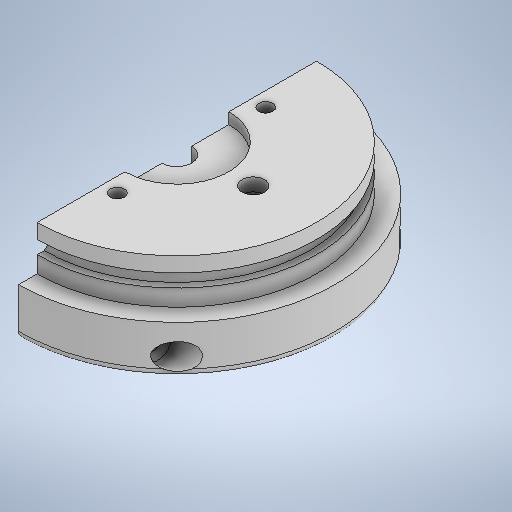
# Autodesk Inventor part: cap2_v0.7.0
Saved by Autodesk Inventor 2025 (Build 290162000, 162)
## iProperties
Created: 2026-01-07
Part Number: cap2_v0.7.0
Material: Generic
Document SubType Name: Modeling
Designer: SLM30
Density: 1 g/cm^3
Appearance: Default
Author: SLM30
Autodesk Inventor part; units mm, degrees
ref_plane "XZ Plane" through (0, 0, 0) normal (0, 1, 0) x (-1, 0, 0)
ref_plane "XY Plane" through (0, 0, 0) normal (0, 0, 1) x (1, 0, 0)
sketch "Sketch4" plane through (0, 0, 0) normal (1, 0, 0) x (0, 1, 0)
  line L0 (0, 0) -> (0, 14)
  line L1 (0, 14) -> (3, 14)
  line L2 (3, 14) -> (3, 37.65)
  line L3 (3, 37.65) -> (-9, 37.65)
  line L4 (-9, 37.65) -> (-9, 42.65)
  line L5 (0, 0) -> (-10, 0)
  line L6 (-10, 0) -> (-10, 15)
  line L7 (-10, 15) -> (-21, 15)
  line L8 (-21, 15) -> (-21, 0)
  line L9 (-21, 0) -> (-29, 0)
  line L10 (-9, 42.65) -> (-21, 42.65)
  line L11 (-21, 42.65) -> (-29, 31.0679)
  line L12 (-29, 31.0679) -> (-29, 0)
  arc A0 (-4.5225, 35.7688) -> (-0.9925, 37.65) centre (-2.7575, 36.7094) ccw
  line L13 (-4.5225, 37.65) -> (-4.5225, 35.7688)
  line L14 (-35.4, 0) -> (9.4, 0) projected
  dimension "d29" = 14
  dimension "d30" = 3
  dimension "d31" = 23.65
  dimension "d32" = 12
  dimension "d33" = 5
  dimension "d34" = 10
  dimension "d35" = 15
  dimension "d36" = 11
  dimension "d37" = 8
  dimension "d38" = 11.5821
  dimension "d39" = 124.634
  dimension "d40" = 3.53
  dimension "d41" = 2
  constraints: 28 end point, 5 perpendicular, 5 vertical, 4 point on line, 2 horizontal, 2 point on circle, 1 centre point
  measures "d29" distance of L0.start L0.end
  measures "d30" distance of L0.end L1.end
  measures "d31" distance of L1.end L2.end
  measures "d32" distance of L2.end L3.end
  measures "d33" distance of L3.end L4.end
  measures "d34" distance of L0.start L5.end
  measures "d35" distance of L5.end L6.end
  measures "d36" distance of L6.end L7.end
  measures "d37" distance of L8.end L9.end
  measures "d38" vertical distance of L10.end L11.end
  measures "d39" angle of L10 L11
  measures "d40" distance of A0.end L13.start
  measures "d41" radius of A0
revolve "Revolution2" add sketch "Sketch4" angle 180 about axis through (0, -10, 0) along (0, 1, 0) contours L5 L6 L7 L8 L9 L12 L11 L10 L4 L3 L13 A0 L2 L1 L0
sketch "Sketch5" plane through (0, 0, 0) normal (0, 1, 0) x (1, 0, 0)
  circle A0 centre (0, 0) radius 4
  dimension "d43" = 8
  constraints: 1 centre point, 1 coincident
  measures "d43" diameter of A0
hole "Hole3" at (0, 0, 0) direction (0, -1, 0) diameter 8 depth 10 tip angle 118
sketch "Sketch6" plane through (0, -29, -31.0679) normal (0, -1, 0) x (1, 0, 0)
  circle A0 centre (0, 31.0679) radius 7
  dimension "d51" = 14
  constraints: 1 centre point, 1 coincident
  measures "d51" diameter of A0
hole "Hole4" at (0, -29, 0) direction (0, 1, 0) diameter 14 depth 8 tip angle 118
sketch "Sketch7" plane through (0, 3, 37.65) normal (0, 1, 0) x (1, 0, 0)
  circle A0 centre (20.601, 37.65) radius 3
  point P0 (0, 37.65)
  dimension "d59" = 6
  dimension "d60" = 20.601
  constraints: 1 centre point
  measures "d59" diameter of A0
  measures "d60" distance of A0.centre point (0, 37.65)
hole "Hole5" at (20.601, 3, 0) direction (0, -1, 0) diameter 6 depth 3.5 tip angle 118
sketch "Sketch8" plane through (0, 3, 37.65) normal (0, 1, 0) x (1, 0, 0)
  circle A0 centre (3.9545, 17.649) radius 1.9085
  line L0 (0, 23.65) -> (0, 0) projected
  point P0 (0, 37.65)
  dimension "d68" = 3.817
  dimension "d69" = 20.001
  dimension "d70" = 3.9545
  constraints: 1 centre point
  measures "d68" diameter of A0
  measures "d69" vertical distance of point (0, 37.65) A0.centre
  measures "d70" distance from line of L0 A0.centre
hole "Hole6" at (3.9545, 3, 20.001) direction (0, -1, 0) diameter 3.817 end through all
mirror "Mirror1" about plane through (0, 0, 0) normal (0, 0, 1) of "Hole6"
sketch "Sketch9" plane through (0, -29, 0) normal (0, -1, 0) x (1, 0, 0)
  circle A0 centre (3.9545, -20.001) radius 1.9085 projected
  circle A1 centre (3.9545, -20.001) radius 4
  point P0 (0, 0)
  dimension "d78" = 8
  constraints: 1 centre point, 1 coincident
  measures "d78" diameter of A1
hole "Hole7" at (3.9545, -29, -20.001) direction (0, 1, 0) diameter 8 depth 4 tip angle 118
mirror "Mirror2" about plane through (0, 0, 0) normal (0, 0, 1) of "Hole7"
sketch "Sketch10" plane through (0, -21, -42.65) normal (-1, 0, 0) x (0, 0, 1)
  circle A0 centre (12.65, 4) radius 1.75
  line L0 (38.65, 11) -> (38.65, 21) projected
  line L1 (28.65, 24) -> (5, 24) projected
  point P0 (42.65, 21)
  dimension "d86" = 3.5
  dimension "d87" = 26
  dimension "d88" = 20
  constraints: 1 centre point
  measures "d86" diameter of A0
  measures "d87" distance from line of L0 A0.centre
  measures "d88" distance from line of A0.centre L1
hole "Hole8" at (0, -17, -30) direction (1, 0, 0) diameter 3.5 end through all
mirror "Mirror3" about plane through (0, 0, 0) normal (0, 0, 1) of "Hole8"
ref_plane "Work Plane1" through (43, 0, 0) normal (1, 0, 0) x (0, 1, 0)
sketch "Sketch11" plane through (43, 0, 0) normal (1, 0, 0) x (0, 1, 0)
  circle A0 centre (-17, 30) radius 1.75 projected
  circle A1 centre (-17, 30) radius 3.5
  point P0 (0, 0)
  dimension "d97" = 7
  constraints: 1 centre point, 1 coincident
  measures "d97" diameter of A1
hole "Hole9" at (43, -17, 30) direction (-1, 0, 0) diameter 7 depth 18 tip angle 118
mirror "Mirror4" about plane through (0, 0, 0) normal (0, 0, 1) of "Hole9"
fillet "Fillet1" radius 2 1 edges at (42.65, -21, 0)
fillet "Fillet2" radius 2 1 edges at (31.0679, -29, 0)
sketch "Sketch12" plane through (0, -21, -15) normal (-1, 0, 0) x (0, 0, 1)
  circle A0 centre (5, 5.5) radius 2.25
  line L0 (0, 0) -> (0, 11) projected
  line L1 (11, 11) -> (0, 11) projected
  point P0 (15, 21)
  dimension "d107" = 4.5
  dimension "d108" = 5
  dimension "d109" = 5.5
  constraints: 1 centre point
  measures "d107" diameter of A0
  measures "d108" distance from line of L0 A0.centre
  measures "d109" distance from line of L1 A0.centre
hole "Hole10" at (0, -15.5, -10) direction (1, 0, 0) diameter 4.5 depth 21.25 tip angle 118
mirror "Mirror5" about plane through (0, 0, 0) normal (0, 0, 1) of "Hole10"
body "Solid2"
